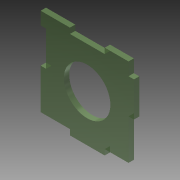
# Autodesk Inventor part: Side B
Saved by Autodesk Inventor 2014 SP2 (Build 180246200, 246)
## iProperties
Created: 2014-11-21
Part Number: Side B
Material: Generic
Document SubType Name: Modeling
Designer: JLM
Density: 1 g/cm^3
Appearance: Default
Author: JLM
Autodesk Inventor part; units mm, degrees
ref_plane "YZ Plane" through (0, 0, 0) normal (1, 0, 0) x (0, 1, 0)
ref_plane "XZ Plane" through (0, 0, 0) normal (0, 1, 0) x (-1, 0, 0)
ref_plane "XY Plane" through (0, 0, 0) normal (0, 0, 1) x (1, 0, 0)
sketch "Sketch1" plane through (0, 0, 0) normal (0, 0, 1) x (1, 0, 0)
  line L0 (-25.5, -25.5) -> (25.5, -25.5)
  line L1 (25.5, -25.5) -> (25.5, 25.5)
  line L2 (25.5, 25.5) -> (-25.5, 25.5)
  line L3 (-25.5, 25.5) -> (-25.5, -25.5)
  line L4 (-25.5, -25.5) -> (25.5, 25.5) construction
  line L5 (25.5, -25.5) -> (-25.5, 25.5) construction
  point P0 (0, 0)
  dimension "d0" = 51
  dimension "d1" = 51
  constraints: 12 end point, 2 midpoint, 2 parallel, 1 horizontal, 1 perpendicular
  measures "d0" distance of L2.end L1.end
  measures "d1" distance of L1.end L0.end
extrude "Extrusion1" add sketch "Sketch1" against normal blind 2.921
sketch "Sketch4" plane through (0, 0, 0) normal (0, 0, 1) x (1, 0, 0)
  line L0 (-25.5, -25.5) -> (-9.5, -25.5)
  line L1 (-9.5, -25.5) -> (-9.5, -22.5)
  line L2 (-9.5, -22.5) -> (-25.5, -22.5)
  line L3 (-25.5, -22.5) -> (-25.5, -25.5)
  line L4 (25.5, 25.5) -> (-25.5, 25.5) projected
  line L5 (-25.5, 25.5) -> (-25.5, -25.5) projected
  line L6 (-25.5, 18.5) -> (-22.5, 18.5)
  line L7 (-22.5, 18.5) -> (-22.5, -0.5)
  line L8 (-22.5, -0.5) -> (-25.5, -0.5)
  line L9 (-25.5, -0.5) -> (-25.5, 18.5)
  line L10 (25.5, -0.5) -> (25.5, 18.5)
  line L11 (-9.5, 25.5) -> (9.5, 25.5)
  line L12 (9.5, 25.5) -> (9.5, 22.5)
  line L13 (9.5, 22.5) -> (-9.5, 22.5)
  line L14 (-9.5, 22.5) -> (-9.5, 25.5)
  line L15 (-25.5, -25.5) -> (25.5, -25.5) projected
  line L16 (25.5, -25.5) -> (25.5, 25.5) projected
  line L17 (25.5, -0.5) -> (22.5, -0.5)
  line L18 (22.5, -0.5) -> (22.5, -22.5)
  line L19 (22.5, -25.5) -> (25.5, -25.5)
  line L20 (25.5, -25.5) -> (25.5, -0.5)
  line L21 (25.5, -25.5) -> (9.5, -25.5)
  line L22 (9.5, -25.5) -> (9.5, -22.5)
  line L23 (9.5, -22.5) -> (22.5, -22.5)
  line L24 (25.5, -22.5) -> (25.5, -25.5)
  line L25 (25.5, 25.5) -> (22.5, 25.5)
  line L26 (22.5, 25.5) -> (22.5, 18.5)
  line L27 (22.5, 18.5) -> (25.5, 18.5)
  line L28 (25.5, 18.5) -> (25.5, 25.5)
  point P0 (0, 0)
  dimension "d16" = 3
  dimension "d37" = 9.5
  dimension "d38" = 16
  dimension "d40" = 3
  dimension "d42" = 19
  dimension "d44" = 3
  dimension "d45" = 19
  dimension "d46" = 16
  dimension "d50" = 25
  dimension "d62" = 3
  dimension "d63" = 25
  dimension "d64" = 3
  dimension "d65" = 19
  dimension "d66" = 16
  dimension "d67" = 3
  dimension "d68" = 7
  dimension "d71" = 19
  dimension "d72" = 7
  constraints: 50 end point, 12 parallel, 6 horizontal, 6 perpendicular, 4 point on line
  measures "d16" distance of L0.end L1.end
  measures "d37" distance from line of point (0, 0) L1
  measures "d38" distance of L0.start L0.end
  measures "d40" distance of L6.start L6.end
  measures "d42" distance of L6.end L7.end
  measures "d44" distance of L13.end L11.start
  measures "d45" distance of L12.end L13.end
  measures "d46" distance between parallel lines of L5 L14
  measures "d50" distance between parallel lines of L0 L8
  measures "d62" distance of L19.start L19.end
  measures "d63" distance between parallel lines of L15 L17
  measures "d64" distance of L24.start L19.end
  measures "d65" distance between parallel lines of L22 L1
  measures "d66" distance between parallel lines of L22 L20
  measures "d67" distance of L4.start L25.end
  measures "d68" distance between parallel lines of L4 L6
  measures "d71" distance between parallel lines of L27 L17
  measures "d72" distance between parallel lines of L4 L27
hole "Hole1" at (-0.1, 0, 0) direction (0, 0, -1) diameter 25.4 end through all
extrude "Extrusion6" cut sketch "Sketch4" against normal up to next contours L3 L2 L1 L0 | L22 L23 L18 L17 L16 L15 | L5 L6 L7 L8 | L4 L12 L13 L14 | L27 L26 L4 L16
equation "\"d1\" = d0"
equation "\"d16\" = d44"
equation "\"d37\" = 0.5 * d45"
equation "\"d38\" = -d37 + 0.5 * d0"
equation "\"d40\" = d44"
equation "\"d42\" = d45"
equation "\"d46\" = -0.5 * d45 + 0.5 * d52"
equation "\"d62\" = d44"
equation "\"d63\" = d50"
equation "\"d64\" = d44"
equation "\"d65\" = d45"
equation "\"d67\" = d44"
equation "\"d71\" = d42"
equation "\"d48\" = 0.5 * d0"
equation "\"d52\" = 51"
body "Solid1"
